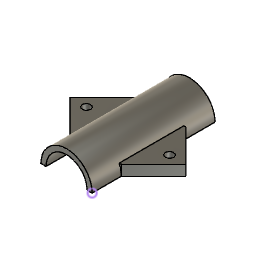
WhirlWax_Assem v1 (Autodesk Fusion 360 archive; units mm, degrees)
design "WeaponWireTunnel"
Autodesk Fusion 360 part; units mm, degrees
note: some values were not read from the file. Set by a fixed rule: which face or edge a step refers to.
sketch "Sketch1" plane through (0, 0, 0) normal (0, 1, 0) x (1, 0, 0)
  circle A0 centre (0, 0) radius 6.35
  circle A1 centre (0, 0) radius 7.9375
  line L0 (7.9375, 0.0011) -> (-7.9375, 0.0011)
  dimension "d1" = 12.7
  dimension "d2" = 15.875
  constraint coincident A0.centre A1.centre
  constraint concentric A0 A1
  constraint coincident A1 L0.start
  constraint coincident A1 L0.end
  constraint horizontal L0
  measures "d1" diameter of A0
  measures "d2" diameter of A1
extrude "Extrude1" add sketch "Sketch1" along normal blind 38.1 contours A0 A1 L0 picked at (7.3788, -0.3944) makes body 1
sketch "Sketch2" plane through (0, 0, 0) normal (0, 0, 1) x (1, 0, 0)
  line L0 (0, 1.0895) -> (-17.9605, 19.05)
  line L1 (-17.9605, 19.05) -> (0, 37.0105)
  line L2 (0, 37.0105) -> (17.9605, 19.05)
  line L3 (17.9605, 19.05) -> (0, 1.0895)
  line L4 (0, 1.0895) -> (0, 37.0105) construction
  line L5 (-17.9605, 19.05) -> (17.9605, 19.05) construction
  line L6 (7.9375, 0) -> (-7.9375, 0) construction
  line L7 (7.9375, 0) -> (7.9375, 38.1) construction
  line L8 (7.9375, 38.1) -> (-7.9375, 38.1) construction
  line L9 (-7.9375, 38.1) -> (-7.9375, 0) construction
  line L10 (0, 38.1) -> (0, 0) construction
  line L11 (-7.9375, 19.05) -> (7.9375, 19.05) construction
  circle A0 centre (-12.8805, 19.05) radius 1.27
  line L12 (-12.8805, 24.13) -> (-12.8805, 13.97) construction
  circle A1 centre (12.8805, 19.05) radius 1.27
  line L13 (7.9375, 9.027) -> (7.9375, 29.073)
  line L14 (-7.9375, 9.027) -> (-7.9375, 29.073)
  point P0 (0, 19.05)
  dimension "d5" = 25.4
  dimension "d6" = 25.4
  dimension "d7" = 2.54
  dimension "d9" = 5.08
  constraint perpendicular L0 L1
  constraint parallel L0 L2
  constraint parallel L1 L3
  constraint coincident L4 P0
  constraint coincident L5 P0
  constraint midpoint L8 L10.start
  constraint coincident L10.end origin
  constraint midpoint L9 L11.start
  constraint midpoint L7 L11.end
  constraint midpoint P0 L11
  constraint parallel L4 L10
  constraint coincident L5 A0.centre
  constraint coincident L1 L12.start
  constraint coincident L0 L12.end
  constraint perpendicular L5 L12
  constraint midpoint A0.centre L12
  constraint symmetric L10 A0 A1
  constraint coincident L7 L13.start
  constraint coincident L3 L13.start
  constraint coincident L2 L13.end
  constraint coincident L7 L13.end
  constraint coincident L9 L14.start
  constraint coincident L0 L14.start
  constraint coincident L9 L14.end
  constraint coincident L1 L14.end
  measures "d5" distance of L0.start L2.end
  measures "d6" distance of L1.end L2.end
  measures "d7" diameter of A0
  measures "d9" distance of L0.end L12
extrude "Extrude2" add sketch "Sketch2" along normal blind 3.175 separate body contours L0 L1 L14 | L2 L3 L13 makes body 2 at (9.1618, 19.05, 0) makes body 3 at (-9.1618, 19.05, 0)
extrude "Extrude3" add 1 faces at (-7.9375, 15.709, 1.0583) along direction (1, 0, 0) up to surface end surface at (7.9276, 25.4, 0.3957) on bodies 1 3 bodies 3 2 1
extrude "Extrude4" add 1 faces at (7.9375, 22.391, 2.1167) along direction (-1, 0, 0) up to surface end surface at (-6.8242, 15.709, 4.0539) on bodies 2 3 bodies 2 3
sketch "Sketch3" plane through (0, 0, 0) normal (0, 1, 0) x (1, 0, 0)
  point P0 (7.9375, 0.0011)

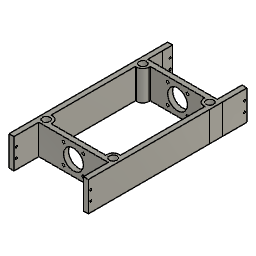
design "WhirlWax_Inside"
Autodesk Fusion 360 part; units mm, degrees
sketch "Sketch1" plane through (0, 0, 0) normal (0, 0, 1) x (1, 0, 0)
  line L0 (101.6, 0) -> (101.6, 203.2)
  line L1 (0, 203.2) -> (0, 0)
  line L2 (95.25, 27.3542) -> (95.25, 31.75)
  line L3 (95.25, 31.75) -> (6.35, 31.75)
  line L4 (6.35, 31.75) -> (6.35, 12.6739)
  line L5 (101.6, 31.75) -> (0, 31.75) construction
  line L6 (0, 31.75) -> (0, 47.625)
  line L7 (0, 47.625) -> (101.6, 47.625) construction
  line L8 (101.6, 47.625) -> (101.6, 31.75)
  circle A0 centre (7.9375, 39.6875) radius 7.9375 construction
  circle A1 centre (7.9375, 39.6875) radius 4.7625
  line L9 (50.8, 31.75) -> (50.8, 47.625)
  circle A2 centre (93.6625, 39.6875) radius 4.7625
  line L10 (0, 101.6) -> (101.6, 101.6)
  line L11 (101.6, 171.45) -> (0, 171.45) construction
  line L12 (95.25, 175.8458) -> (95.25, 171.45)
  line L13 (95.25, 171.45) -> (6.35, 171.45)
  line L14 (6.35, 171.45) -> (6.35, 190.5261)
  line L15 (101.6, 155.575) -> (101.6, 171.45)
  line L16 (0, 155.575) -> (101.6, 155.575) construction
  line L17 (0, 171.45) -> (0, 155.575)
  circle A3 centre (7.9375, 163.5125) radius 4.7625
  circle A4 centre (93.6625, 163.5125) radius 4.7625
  line L18 (95.25, 47.625) -> (6.35, 47.625)
  line L19 (6.35, 47.625) -> (6.35, 155.575)
  line L20 (6.35, 155.575) -> (95.25, 155.575)
  line L21 (95.25, 155.575) -> (95.25, 47.625)
  line L22 (6.35, 12.6739) -> (6.35, 0)
  line L23 (95.25, 27.3542) -> (95.25, 0)
  line L24 (0, 0) -> (6.35, 0)
  line L25 (95.25, 0) -> (101.6, 0)
  line L26 (6.35, 190.5261) -> (6.35, 203.2)
  line L27 (95.25, 175.8458) -> (95.25, 203.2)
  line L28 (101.6, 203.2) -> (95.25, 203.2)
  line L29 (6.35, 203.2) -> (0, 203.2)
  circle A5 centre (7.9375, 163.5125) radius 7.9375 construction
  circle A6 centre (93.6625, 163.5125) radius 7.9375 construction
  arc A7 (85.725, 163.5123) -> (93.6625, 155.575) centre (93.6625, 163.5125) ccw
  arc A8 (7.9421, 155.575) -> (15.875, 163.5125) centre (7.9375, 163.5125) ccw
  line L30 (85.8854, 165.1) -> (15.7146, 165.1) construction
  line L31 (15.875, 163.5125) -> (15.875, 165.1)
  line L32 (15.875, 165.1) -> (85.7183, 165.1)
  line L33 (85.7183, 165.1) -> (85.725, 163.5123)
  line L34 (15.875, 38.1) -> (85.7183, 38.1)
  line L35 (85.7183, 38.1) -> (85.725, 39.6877)
  line L36 (15.875, 39.6875) -> (15.875, 38.1)
  arc A9 (15.875, 39.6875) -> (7.9421, 47.625) centre (7.9375, 39.6875) ccw
  arc A10 (93.6625, 47.625) -> (85.725, 39.6877) centre (93.6625, 39.6875) ccw
  dimension "d1" = 101.6
  dimension "d2" = 203.2
  dimension "d4" = 6.35
  dimension "d5" = 6.35
  dimension "d7" = 15.875
  dimension "d8" = 9.525
  dimension "d10" = 6.35
  dimension "d11" = 6.35
  dimension "d23" = 31.75
  dimension "d24" = 6.35
  constraint horizontal L24
  constraint vertical L0
  constraint horizontal L28
  constraint vertical L1
  constraint coincident L1.end L24.start
  constraint vertical L2
  constraint horizontal L3
  constraint vertical L4
  constraint horizontal L5
  constraint vertical L6
  constraint horizontal L7
  constraint vertical L8
  constraint coincident L1 L6.end
  constraint coincident L0 L5.start
  constraint tangent L5 A0
  constraint tangent L7 A0
  constraint tangent L6 A0
  constraint concentric A0 A1
  constraint midpoint L5 L9.start
  constraint midpoint L7 L9.end
  constraint symmetric A1 L9 A2
  constraint midpoint L1 L10.start
  constraint midpoint L0 L10.end
  constraint symmetric L4.end L10 L14.end
  constraint symmetric L2.start L10 L12.start
  constraint symmetric L2.end L10 L12.end
  constraint symmetric L3.end L10 L13.end
  constraint symmetric L5.start L10 L11.start
  constraint symmetric L5.end L10 L11.end
  constraint symmetric L6.end L10 L16.start
  constraint symmetric L7.end L10 L15.start
  constraint symmetric A1 L10 A3
  constraint symmetric A2 L10 A4
  constraint horizontal L18
  constraint vertical L19
  constraint horizontal L20
  constraint vertical L21
  constraint coincident L16 L19.end
  constraint coincident L7 L18.start
  constraint coincident L2.end L5
  constraint perpendicular L22 L24
  constraint coincident L23.end L24
  constraint perpendicular L23 L24
  constraint collinear L24 L25
  constraint coincident L26.end L28
  constraint perpendicular L26 L28
  constraint perpendicular L27 L28
  constraint collinear L28 L29
  constraint tangent L13 A5
  constraint tangent L11 A6
  constraint coincident A6 A7.end
  constraint coincident L20 A7.end
  constraint coincident A4.centre A6.centre
  constraint coincident A5 A8.end
  constraint coincident A5 A8.start
  constraint coincident L20 A8.start
  constraint coincident A3.centre A5.centre
  constraint coincident A6 L30.start
  constraint coincident A5 L30.end
  constraint coincident L30 L31.end
  constraint perpendicular L30 L31
  constraint coincident L30 L32.end
  constraint symmetric L10 A7.start L35.end
  constraint symmetric L10 A7.end A10.start
  constraint symmetric L10 A7 A10
  constraint symmetric L10 A8.start A9.end
  constraint symmetric L10 A8.end L36.start
  constraint symmetric L10 A8 A9
  constraint symmetric L10 L31.end L34.start
  constraint symmetric L10 L32.end L34.end
  constraint coincident A2.centre A10.centre
  measures "d1" distance of L1.end L0.start
  measures "d2" distance of L1.end L1.start
  measures "d4" distance of L0 L2
  measures "d5" distance of L1 L4
  measures "d7" distance of L5 L7
  measures "d8" diameter of A1
  measures "d10" distance of L1 L19
  measures "d11" distance of L0 L21
  measures "d23" distance of L5 L22.end
  measures "d24" distance of L13 L30
extrude "Extrude1" add sketch "Sketch1" along normal blind 38.1 contours L0 L2 L3 L8 L9 L10 L18 L21 L23 L25 L34 L35 A10 | L0 L1 L10 L12 L13 L14 L15 L17 L19 L20 L21 L26 L27 L28 L29 A7 A8 L31 L32 L33 | L1 L3 L4 L6 L9 L10 L18 L19 L22 L24 L34 L36 A9
sketch "Sketch2" plane through (0, 155.575, 0) normal (0, -1, 0) x (1, 0, 0)
  line L0 (93.6625, 0) -> (95.25, 0)
  line L1 (95.25, 0) -> (95.25, 38.1)
  line L2 (95.25, 38.1) -> (93.6625, 38.1)
  line L3 (6.35, 38.1) -> (6.35, 0)
  circle A0 centre (63.4966, 31.75) radius 1.7272
  circle A1 centre (38.0966, 31.75) radius 1.7272
  circle A2 centre (38.0966, 6.35) radius 1.7272
  circle A3 centre (63.4966, 6.35) radius 1.7272
  circle A4 centre (50.7966, 19.05) radius 7.1 construction
  circle A5 centre (50.7966, 19.05) radius 12.7
  line L4 (93.6625, 38.1) -> (93.6625, 0)
  line L5 (6.35, 0) -> (7.9421, 0)
  line L6 (7.9421, 0) -> (7.9421, 38.1)
  line L7 (7.9421, 38.1) -> (6.35, 38.1)
  line L8 (15.875, 0) -> (85.7183, 0)
  line L9 (15.875, 38.1) -> (85.7183, 38.1)
  line L10 (63.4966, 31.75) -> (63.4966, 6.35) construction
  line L11 (63.4966, 6.35) -> (38.0966, 6.35) construction
  line L12 (38.0966, 6.35) -> (38.0966, 31.75) construction
  line L13 (38.0966, 31.75) -> (63.4966, 31.75) construction
  line L14 (50.7966, 38.1) -> (50.7966, 0)
  dimension "d18" = 25.4
  constraint concentric A4 A5
  constraint coincident A0.centre L10.start
  constraint coincident A3.centre L10.end
  constraint vertical L10
  constraint coincident A2.centre L11.end
  constraint perpendicular L10 L11
  constraint coincident A1.centre L12.end
  constraint perpendicular L11 L12
  constraint perpendicular L10 L13
  constraint tangent A5 L11
  constraint tangent A5 L10
  constraint tangent A5 L13
  constraint tangent A5 L12
  constraint midpoint L9 L14.start
  constraint midpoint L8 L14.end
  constraint coincident A4.centre L14
  measures "d18" diameter of A5
extrude "Extrude2" cut sketch "Sketch2" along normal up to surface (-15.875 mm away) and the other way up to surface (-123.825 mm away) contours A0 | A1 | A2 | A3 | A5 L14 | A5 L14
sketch "Sketch3" plane through (0, 0, 0) normal (-1, 0, 0) x (0, -1, 0)
  line L0 (-155.575, 0) -> (0, 0)
  line L1 (0, 0) -> (0, 38.1)
  line L2 (0, 38.1) -> (-155.575, 38.1)
  line L3 (-155.575, 38.1) -> (-155.575, 0)
  circle A0 centre (-3.175, 12.7) radius 1.27
  circle A1 centre (-3.175, 25.4) radius 1.27
  line L4 (-47.625, 38.1) -> (-155.575, 38.1)
  line L5 (-101.6, 38.1) -> (-101.6, 0)
  circle A2 centre (-200.025, 12.7) radius 1.27
  circle A3 centre (-200.025, 25.4) radius 1.27
  dimension "d25" = 2.54
  dimension "d26" = 2.54
  dimension "d27" = 12.7
  dimension "d28" = 12.7
  dimension "d29" = 3.175
  dimension "d30" = 3.175
  constraint midpoint L4 L5.start
  constraint coincident L0 L5.end
  constraint perpendicular L0 L5
  constraint symmetric A0 L5 A2
  constraint symmetric A1 L5 A3
  measures "d25" diameter of A0
  measures "d26" diameter of A1
  measures "d27" distance of L2 A1.centre
  measures "d28" distance of L0 A0.centre
  measures "d29" distance of L1 A0.centre
  measures "d30" distance of L1 A1.centre
extrude "Extrude3" cut sketch "Sketch3" along normal through all and the other way through all contours A0 | A1 | A2 | A3
sketch "Sketch4" plane through (0, 38.1, 0) normal (0, 1, 0) x (-1, 0, 0)
  circle A0 centre (-50.7966, 19.05) radius 12.7
  circle A1 centre (-38.0966, 6.35) radius 1.7272
  circle A2 centre (-63.4966, 31.75) radius 1.7272
  circle A3 centre (-38.0966, 31.75) radius 1.7272
  circle A4 centre (-63.4966, 6.35) radius 1.7272
  line L0 (-85.7183, 0) -> (-15.875, 0)
  line L1 (-15.875, 0) -> (-15.875, 38.1)
  line L2 (-15.875, 38.1) -> (-85.7183, 38.1)
  line L3 (-85.7183, 38.1) -> (-85.7183, 0)
  line L4 (-95.25, 0) -> (-95.25, 38.1)
  circle A5 centre (-86.36, 0) radius 5.715
  circle A6 centre (-86.36, 0) radius 8.89
  circle A7 centre (-50.7966, 19.05) radius 30.1625 construction
  dimension "d33" = 17.78
  dimension "d34" = 60.325
  dimension "d35" = 11.43
  constraint coincident L0 A5.centre
  constraint concentric A5 A6
  constraint concentric A0 A7
  constraint tangent L4 A6
  measures "d33" diameter of A6
  measures "d34" diameter of A7
  measures "d35" diameter of A5
extrude "Extrude4" cut sketch "Sketch4" against normal blind 6.35 contours L0 L3 A5 picked at (-85.4455, 3.7347)
equation "d34 = 2 in + ( 3 / 8 ) * 1 in"

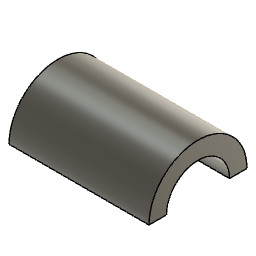
design "lilTunnel"
Autodesk Fusion 360 part; units mm, degrees
sketch "Sketch1" plane through (0, 0, 0) normal (1, 0, 0) x (0, 1, 0)
  line L0 (0, 0) -> (101.6, 0) construction
  line L1 (101.6, 0) -> (101.6, 38.1) construction
  line L2 (101.6, 38.1) -> (0, 38.1) construction
  line L3 (0, 38.1) -> (0, 0) construction
  circle A0 centre (50.8, 19.05) radius 30.1625 construction
  line L4 (101.6, 0) -> (85.725, 0) construction
  line L5 (85.725, 15.875) -> (101.6, 15.875) construction
  line L6 (101.6, 15.875) -> (101.6, 0) construction
  arc A1 (86.36, 5.715) -> (80.645, 0) centre (86.36, 0) ccw
  arc A2 (86.36, 8.89) -> (77.47, 0) centre (86.36, 0) ccw
  line L7 (86.36, 8.89) -> (86.36, 5.715)
  line L8 (77.47, 0) -> (80.645, 0)
  line L9 (101.6, 38.1) -> (95.25, 38.1) construction
  line L10 (95.25, 38.1) -> (95.25, -0.2036) construction
  line L11 (95.25, -0.2036) -> (101.6, -0.2036) construction
  line L12 (101.6, -0.2036) -> (101.6, 38.1) construction
  arc A3 (92.075, 0) -> (86.36, 5.715) centre (86.36, 0) ccw
  arc A4 (95.25, 0) -> (86.36, 8.89) centre (86.36, 0) ccw
  line L13 (92.075, 0) -> (95.25, 0)
  dimension "d1" = 101.6
  dimension "d2" = 38.1
  dimension "d3" = 60.325
  dimension "d4" = 15.875
  dimension "d5" = 15.875
  dimension "d8" = 6.35
  dimension "d12" = 50.8
  dimension "d13" = 5.715
  dimension "d14" = 8.89
  constraint horizontal L0
  constraint vertical L1
  constraint horizontal L2
  constraint vertical L3
  constraint coincident L0.start L3.end
  constraint horizontal L4
  constraint horizontal L5
  constraint vertical L6
  constraint coincident L0 A1.end
  constraint coincident L0 A2.end
  constraint horizontal L9
  constraint vertical L10
  constraint horizontal L11
  constraint vertical L12
  constraint coincident L10 A4.start
  measures "d1" distance of L0.start L0.end
  measures "d2" distance of L0.start L2.end
  measures "d3" diameter of A0
  measures "d4" distance of L0.end L4.end
  measures "d5" distance of L0.end L5.end
  measures "d8" distance of L1.end L9.end
  measures "d12" distance of L3 A0.centre
  measures "d13" radius of A3
  measures "d14" radius of A4
extrude "Extrude1" add sketch "Sketch1" along normal blind 25.4
equation "d3 = 2 3/8\""

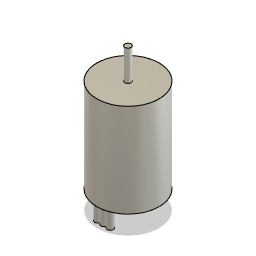
design "2030 motor"
Autodesk Fusion 360 part; units mm, degrees
sketch "Sketch1" plane through (0, 0, 0) normal (0, 1, 0) x (1, 0, 0)
  circle A0 centre (0, -2.6241) radius 10
  dimension "d1" = 20
  measures "d1" diameter of A0
extrude "Extrude1" add sketch "Sketch1" along normal blind 30 makes body 1
sketch "Sketch2" plane through (0, 30, 0) normal (0, 1, 0) x (-1, 0, 0)
  circle A0 centre (0, 2.6241) radius 10
  circle A1 centre (0, 2.6241) radius 1
  dimension "d4" = 2
  constraint concentric A0 A1
  measures "d4" diameter of A1
extrude "Extrude2" add sketch "Sketch2" along normal blind 9.8 contours A1 bodies 1
sketch "Sketch3" plane through (0, 0, 0) normal (0, -1, 0) x (1, 0, 0)
  circle A0 centre (0, 2.6241) radius 10
  circle A1 centre (-2, 10.3376) radius 1
  circle A2 centre (0, 10.3376) radius 1
  circle A3 centre (2, 10.3376) radius 1
  dimension "d7" = 2
  dimension "d8" = 2
  dimension "d9" = 2
  dimension "d10" = 2
  dimension "d11" = 2
  constraint horizontal A2.centre A3.centre
  constraint horizontal A1.centre A2.centre
  measures "d7" diameter of A1
  measures "d8" diameter of A2
  measures "d9" diameter of A3
  measures "d10" distance of A1.centre A2.centre
  measures "d11" distance of A2.centre A3.centre
extrude "Extrude3" add sketch "Sketch3" along normal blind 6 separate body contours A1 | A3 | A2 makes body 2
combine "Combine1" operation add target body 2 tool bodies 1

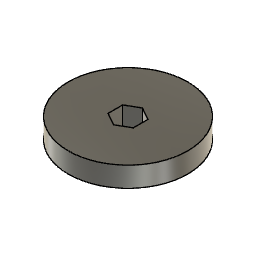
design "Basic_Wheel"
Autodesk Fusion 360 part; units mm, degrees
sketch "Sketch1" plane through (0, 0, 0) normal (0, 0, 1) x (1, 0, 0)
  circle A0 centre (0, 0) radius 30.1625
  line L0 (6.35, 3.6662) -> (0, 7.3323)
  line L1 (0, 7.3323) -> (-6.35, 3.6662)
  line L2 (-6.35, 3.6662) -> (-6.35, -3.6662)
  line L3 (-6.35, -3.6662) -> (0, -7.3323)
  line L4 (0, -7.3323) -> (6.35, -3.6662)
  line L5 (6.35, -3.6662) -> (6.35, 3.6662)
  dimension "d1" = 60.325
  dimension "d5" = 6.35
  constraint coincident A0.centre origin
  measures "d1" diameter of A0
  measures "d5" distance of A0.centre L5
extrude "Extrude1" add sketch "Sketch1" along normal blind 10.16
equation "d1 = 2 in + ( 3 / 8 ) * 1 in"

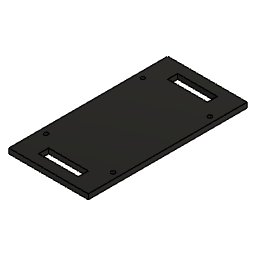
design "WhirlWax_TopPlate"
Autodesk Fusion 360 part; units mm, degrees
sketch "Sketch1" plane through (0, 0, 0) normal (0, 0, 1) x (1, 0, 0)
  line L0 (101.6, 203.2) -> (0, 203.2)
  line L1 (101.6, 203.2) -> (101.6, 0)
  line L2 (0, 0) -> (0, 203.2)
  line L3 (0, 0) -> (101.6, 0)
  dimension "d37" = 203.2
  dimension "d38" = 101.6
  constraint horizontal L0
  constraint perpendicular L0 L2
  constraint coincident L2.start L3.start
  constraint perpendicular L1 L3
  constraint parallel L0 L3
  measures "d37" distance of L0.end L2.start
  measures "d38" distance of L2.start L1.end
extrude "Extrude1" add sketch "Sketch1" along normal blind 6.35
sketch "Sketch2" plane through (0, 0, 0) normal (0, 1, 0) x (1, 0, 0)
  line L0 (0, -3.175) -> (76.2, -3.175) construction
  line L1 (76.2, -3.175) -> (76.2, -41.275) construction
  line L2 (76.2, -41.275) -> (0, -41.275) construction
  line L3 (0, -41.275) -> (0, -3.175) construction
  line L4 (38.1, -41.275) -> (38.1, -3.175) construction
  line L5 (76.2, -22.225) -> (0, -22.225) construction
  circle A0 centre (38.1, -22.225) radius 23.8125
  point P0 (101.6, -6.35)
  dimension "d6" = 47.625
  dimension "d32" = 38.1
  constraint horizontal L0
  constraint vertical L1
  constraint horizontal L2
  constraint vertical L3
  constraint midpoint L2 L4.start
  constraint midpoint L0 L4.end
  constraint midpoint L1 L5.start
  constraint midpoint L3 L5.end
  constraint midpoint L4 A0.centre
  measures "d6" diameter of A0
  measures "d32" distance of L0.end L1.end
sketch "Sketch3" plane through (0, 0, 6.35) normal (0, 0, 1) x (-1, 0, 0)
  line L0 (-101.6, 0) -> (-101.6, -203.2)
  line L1 (0, -203.2) -> (0, 0)
  line L2 (0, 0) -> (-101.6, 0) construction
  line L3 (-61.9125, 0) -> (-14.2875, 0) construction
  line L4 (0, -31.75) -> (-101.6, -31.75)
  line L5 (-101.6, -31.75) -> (-101.6, -47.625)
  line L6 (-101.6, -47.625) -> (0, -47.625)
  line L7 (0, -47.625) -> (0, -31.75)
  circle A0 centre (-93.6625, -39.6875) radius 7.9375 construction
  circle A1 centre (-93.6625, -39.6875) radius 4.7625
  circle A2 centre (-93.6625, -39.6875) radius 2.54
  line L8 (-50.8, -203.2) -> (-50.8, 0) construction
  line L9 (-50.8, -101.6) -> (-8.4033, -101.6)
  line L10 (-101.6, -155.575) -> (0, -155.575)
  line L11 (0, -171.45) -> (-101.6, -171.45)
  circle A3 centre (-93.6625, -163.5125) radius 4.7625
  line L12 (-101.6, -171.45) -> (-101.6, -155.575)
  line L13 (0, -155.575) -> (0, -171.45)
  circle A4 centre (-93.6625, -163.5125) radius 2.54
  line L14 (-25.4, -190.5) -> (-76.2, -190.5)
  line L15 (-76.2, -190.5) -> (-76.2, -177.8)
  line L16 (-76.2, -177.8) -> (-25.4, -177.8)
  line L17 (-25.4, -177.8) -> (-25.4, -190.5)
  line L18 (0, 0) -> (-101.6, 0)
  circle A5 centre (-7.9375, -163.5125) radius 4.7625
  circle A6 centre (-7.9375, -163.5125) radius 2.54
  circle A7 centre (-7.9375, -39.6875) radius 4.7625
  circle A8 centre (-7.9375, -39.6875) radius 2.54
  line L19 (-76.2, -12.7) -> (-76.2, -25.4)
  line L20 (-76.2, -25.4) -> (-25.4, -25.4)
  line L21 (-25.4, -12.7) -> (-76.2, -12.7)
  line L22 (-25.4, -25.4) -> (-25.4, -12.7)
  line L23 (-101.6, -203.2) -> (0, -203.2)
  point P0 (-93.6625, -163.5125)
  dimension "d25" = 15.875
  dimension "d26" = 9.525
  dimension "d27" = 5.08
  dimension "d29" = 12.7
  dimension "d30" = 25.4
  dimension "d31" = 25.4
  dimension "d36" = 6.35
  dimension "d39" = 12.7
  constraint coincident L1.end L2.start
  constraint coincident L0.start L2.end
  constraint horizontal L4
  constraint vertical L5
  constraint horizontal L6
  constraint vertical L7
  constraint coincident L1 L4.start
  constraint tangent L4 A0
  constraint tangent L5 A0
  constraint tangent L6 A0
  constraint concentric A0 A1
  constraint concentric A1 A2
  constraint midpoint L8 L9.start
  constraint symmetric L4.start L9 L11.start
  constraint symmetric L4.end L9 L11.end
  constraint symmetric L5.end L9 L10.start
  constraint symmetric L6.end L9 L10.end
  constraint symmetric A1 L9 A3
  constraint symmetric A0.centre L9 P0
  constraint symmetric A2 L9 A4
  constraint horizontal L14
  constraint vertical L15
  constraint horizontal L16
  constraint vertical L17
  constraint coincident L0 L5.end
  constraint horizontal L9
  constraint symmetric A1 L8 A7
  constraint symmetric A2 L8 A8
  constraint symmetric L8 A3 A5
  constraint symmetric L8 A4 A6
  constraint symmetric L9 L14.start L21.start
  constraint symmetric L9 L14.end L19.start
  constraint symmetric L9 L15.end L19.end
  constraint symmetric L9 L16.end L20.end
  constraint midpoint L18 L8.end
  constraint midpoint L8.start L23
  measures "d25" distance of L4.start L6.end
  measures "d26" diameter of A1
  measures "d27" diameter of A2
  measures "d29" distance of L14.start L16.end
  measures "d30" distance of L1 L17
  measures "d31" distance of L0 L15
  measures "d36" distance of L11 L16
  measures "d39" distance of L14 L23
extrude "Extrude6" cut sketch "Sketch3" along normal through all and the other way through all contours A2 | A4 | L14 L15 L16 L17 | A6 | A8 | L19 L20 L21 L22
equation "d6 = 1 in + ( 7 / 8 ) * 1 in"

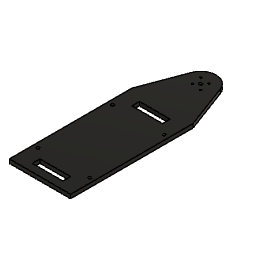
design "WhirlWax_Plate_D3536"
Autodesk Fusion 360 part; units mm, degrees
sketch "Sketch1" plane through (0, 0, 0) normal (0, 0, 1) x (1, 0, 0)
  line L0 (101.6, 203.2) -> (0, 203.2)
  line L1 (101.6, 203.2) -> (101.6, 0)
  line L2 (0, 0) -> (0, 203.2)
  line L3 (0, 0) -> (101.6, 0)
  dimension "d37" = 203.2
  dimension "d38" = 101.6
  constraint horizontal L0
  constraint perpendicular L0 L2
  constraint coincident L2.start L3.start
  constraint perpendicular L1 L3
  constraint parallel L0 L3
  measures "d37" distance of L0.end L2.start
  measures "d38" distance of L2.start L1.end
extrude "Extrude1" add sketch "Sketch1" along normal blind 6.35
sketch "Sketch2" plane through (0, 0, 0) normal (0, 1, 0) x (1, 0, 0)
  line L0 (0, -3.175) -> (76.2, -3.175) construction
  line L1 (76.2, -3.175) -> (76.2, -41.275) construction
  line L2 (76.2, -41.275) -> (0, -41.275) construction
  line L3 (0, -41.275) -> (0, -3.175) construction
  line L4 (38.1, -41.275) -> (38.1, -3.175) construction
  line L5 (76.2, -22.225) -> (0, -22.225) construction
  circle A0 centre (38.1, -22.225) radius 23.8125
  point P0 (101.6, -6.35)
  dimension "d6" = 47.625
  dimension "d32" = 38.1
  constraint horizontal L0
  constraint vertical L1
  constraint horizontal L2
  constraint vertical L3
  constraint midpoint L2 L4.start
  constraint midpoint L0 L4.end
  constraint midpoint L1 L5.start
  constraint midpoint L3 L5.end
  constraint midpoint L4 A0.centre
  measures "d6" diameter of A0
  measures "d32" distance of L0.end L1.end
sketch "Sketch3" plane through (0, 0, 6.35) normal (0, 0, 1) x (-1, 0, 0)
  line L0 (-101.6, 0) -> (-101.6, -203.2)
  line L1 (0, -203.2) -> (0, 0)
  line L2 (0, 0) -> (-101.6, 0) construction
  line L3 (-61.9125, 0) -> (-14.2875, 0) construction
  line L4 (0, -31.75) -> (-101.6, -31.75)
  line L5 (-101.6, -31.75) -> (-101.6, -47.625)
  line L6 (-101.6, -47.625) -> (0, -47.625)
  line L7 (0, -47.625) -> (0, -31.75)
  circle A0 centre (-93.6625, -39.6875) radius 7.9375 construction
  circle A1 centre (-93.6625, -39.6875) radius 4.7625
  circle A2 centre (-93.6625, -39.6875) radius 2.54
  line L8 (-50.8, -203.2) -> (-50.8, 0) construction
  line L9 (-50.8, -101.6) -> (-8.4033, -101.6)
  line L10 (-101.6, -155.575) -> (0, -155.575)
  line L11 (0, -171.45) -> (-101.6, -171.45)
  circle A3 centre (-93.6625, -163.5125) radius 4.7625
  line L12 (-101.6, -171.45) -> (-101.6, -155.575)
  line L13 (0, -155.575) -> (0, -171.45)
  circle A4 centre (-93.6625, -163.5125) radius 2.54
  line L14 (-25.4, -190.5) -> (-76.2, -190.5)
  line L15 (-76.2, -190.5) -> (-76.2, -177.8)
  line L16 (-76.2, -177.8) -> (-25.4, -177.8)
  line L17 (-25.4, -177.8) -> (-25.4, -190.5)
  line L18 (0, 0) -> (-101.6, 0)
  circle A5 centre (-7.9375, -163.5125) radius 4.7625
  circle A6 centre (-7.9375, -163.5125) radius 2.54
  circle A7 centre (-7.9375, -39.6875) radius 4.7625
  circle A8 centre (-7.9375, -39.6875) radius 2.54
  line L19 (-76.2, -12.7) -> (-76.2, -25.4)
  line L20 (-76.2, -25.4) -> (-25.4, -25.4)
  line L21 (-25.4, -12.7) -> (-76.2, -12.7)
  line L22 (-25.4, -25.4) -> (-25.4, -12.7)
  line L23 (-101.6, -203.2) -> (0, -203.2)
  point P0 (-93.6625, -163.5125)
  dimension "d25" = 15.875
  dimension "d26" = 9.525
  dimension "d27" = 5.08
  dimension "d29" = 12.7
  dimension "d30" = 25.4
  dimension "d31" = 25.4
  dimension "d36" = 6.35
  dimension "d39" = 12.7
  constraint coincident L1.end L2.start
  constraint coincident L0.start L2.end
  constraint horizontal L4
  constraint vertical L5
  constraint horizontal L6
  constraint vertical L7
  constraint coincident L1 L4.start
  constraint tangent L4 A0
  constraint tangent L5 A0
  constraint tangent L6 A0
  constraint concentric A0 A1
  constraint concentric A1 A2
  constraint midpoint L8 L9.start
  constraint symmetric L4.start L9 L11.start
  constraint symmetric L4.end L9 L11.end
  constraint symmetric L5.end L9 L10.start
  constraint symmetric L6.end L9 L10.end
  constraint symmetric A1 L9 A3
  constraint symmetric A0.centre L9 P0
  constraint symmetric A2 L9 A4
  constraint horizontal L14
  constraint vertical L15
  constraint horizontal L16
  constraint vertical L17
  constraint coincident L0 L5.end
  constraint horizontal L9
  constraint symmetric A1 L8 A7
  constraint symmetric A2 L8 A8
  constraint symmetric L8 A3 A5
  constraint symmetric L8 A4 A6
  constraint symmetric L9 L14.start L21.start
  constraint symmetric L9 L14.end L19.start
  constraint symmetric L9 L15.end L19.end
  constraint symmetric L9 L16.end L20.end
  constraint midpoint L18 L8.end
  constraint midpoint L8.start L23
  measures "d25" distance of L4.start L6.end
  measures "d26" diameter of A1
  measures "d27" diameter of A2
  measures "d29" distance of L14.start L16.end
  measures "d30" distance of L1 L17
  measures "d31" distance of L0 L15
  measures "d36" distance of L11 L16
  measures "d39" distance of L14 L23
extrude "Extrude6" cut sketch "Sketch3" along normal through all and the other way through all contours A2 | A4 | L14 L15 L16 L17 | A6 | A8 | L19 L20 L21 L22
sketch "Sketch5" plane through (0, 0, 6.35) normal (0, 0, 1) x (-1, 0, 0)
  circle A0 centre (-93.6625, -39.6875) radius 2.54
  circle A1 centre (-93.6625, -163.5125) radius 2.54
  circle A2 centre (-7.9375, -39.6875) radius 2.54
  circle A3 centre (-7.9375, -163.5125) radius 2.54
  line L0 (-25.4, -177.8) -> (-25.4, -190.5)
  line L1 (-25.4, -190.5) -> (-76.2, -190.5)
  line L2 (-76.2, -190.5) -> (-76.2, -177.8)
  line L3 (-76.2, -177.8) -> (-25.4, -177.8)
  line L4 (-25.4, -25.4) -> (-76.2, -25.4)
  line L5 (-76.2, -25.4) -> (-76.2, -12.7)
  line L6 (-76.2, -12.7) -> (-25.4, -12.7)
  line L7 (-25.4, -12.7) -> (-25.4, -25.4)
  line L8 (-101.6, -203.2) -> (0, -203.2)
  line L9 (0, -203.2) -> (0, 0)
  line L10 (0, 0) -> (-101.6, 0)
  line L11 (-101.6, 0) -> (-101.6, -203.2)
  line L12 (-50.8, -203.2) -> (-50.8, -292.1) construction
  circle A4 centre (-50.8, -266.7) radius 25.4
  line L13 (-101.6, -203.2) -> (-74.5978, -275.5783)
  line L14 (0, -203.2) -> (-27.0022, -275.5783)
  circle A5 centre (-44.0825, -259.9825) radius 1.5
  circle A6 centre (-57.5175, -273.4175) radius 1.5
  line L15 (-57.5175, -273.4175) -> (-44.0825, -259.9825) construction
  circle A7 centre (-41.9612, -275.5388) radius 1.5
  circle A8 centre (-59.6388, -257.8612) radius 1.5
  line L16 (-41.9612, -275.5388) -> (-59.6388, -257.8612) construction
  circle A9 centre (-50.8, -266.7) radius 2.54
  point P0 (-50.8, -266.7)
  dimension "d40" = 25.4
  dimension "d43" = 3
  dimension "d44" = 3
  dimension "d45" = 19
  dimension "d46" = 3
  dimension "d47" = 3
  dimension "d48" = 25
  dimension "d49" = 135
  dimension "d52" = 63.5
  constraint midpoint L8 L12.start
  constraint perpendicular L8 L12
  constraint coincident L12 P0
  constraint coincident L12.end A4
  constraint coincident L8.start L11.end
  constraint coincident A4 L13.end
  constraint tangent A4 L13
  constraint coincident L8.end L9.start
  constraint coincident A4 L14.end
  constraint tangent A4 L14
  constraint coincident A6.centre L15.start
  constraint coincident A5.centre L15.end
  constraint coincident A7.centre L16.start
  constraint coincident A8.centre L16.end
  constraint perpendicular L15 L16
  constraint midpoint L15 L16
  constraint midpoint L16 P0
  constraint coincident P0 A4.centre
  measures "d40" distance of L12.end P0
  measures "d43" diameter of A5
  measures "d44" diameter of A6
  measures "d45" distance of A6.centre A5.centre
  measures "d46" diameter of A7
  measures "d47" diameter of A8
  measures "d48" distance of A7.centre A8.centre
  measures "d49" angle of L12 L16
  measures "d52" distance of L12.start P0
extrude "Extrude7" add sketch "Sketch5" against normal blind 6.35 contours L8 A4 L13 L14 | A4
equation "d6 = 1 in + ( 7 / 8 ) * 1 in"

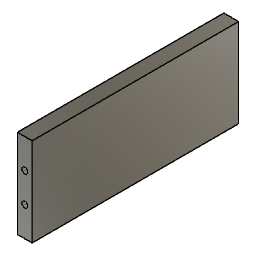
design "WhirlWax_WheelGuardNoTunnel"
Autodesk Fusion 360 part; units mm, degrees
sketch "Sketch1" plane through (0, 0, 0) normal (1, 0, 0) x (0, 1, 0)
  line L0 (0, 0) -> (88.9, 0)
  line L1 (88.9, 0) -> (88.9, 38.1)
  line L2 (88.9, 38.1) -> (0, 38.1)
  line L3 (0, 38.1) -> (0, 0)
  dimension "d1" = 88.9
  dimension "d2" = 38.1
  constraint horizontal L0
  constraint vertical L1
  constraint horizontal L2
  constraint vertical L3
  constraint coincident L0.start L3.end
  measures "d1" distance of L0.start L0.end
  measures "d2" distance of L0.start L2.end
extrude "Extrude1" add sketch "Sketch1" along normal blind 6.35
sketch "Sketch2" plane through (0, 0, 0) normal (0, -1, 0) x (1, 0, 0)
  line L0 (0, 38.1) -> (0, 0)
  line L1 (0, 0) -> (6.35, 0)
  line L2 (6.35, 0) -> (6.35, 38.1)
  line L3 (6.35, 38.1) -> (0, 38.1)
  line L4 (3.175, 38.1) -> (3.175, 0) construction
  circle A0 centre (3.175, 25.4) radius 1.27
  circle A1 centre (3.175, 12.7) radius 1.27
  dimension "d5" = 2.54
  dimension "d6" = 2.54
  dimension "d7" = 12.7
  dimension "d8" = 12.7
  constraint midpoint L3 L4.start
  constraint midpoint L1 L4.end
  constraint coincident L4 A0.centre
  constraint coincident L4 A1.centre
  measures "d5" diameter of A0
  measures "d6" diameter of A1
  measures "d7" distance of L1 A1.centre
  measures "d8" distance of L3 A0.centre
extrude "Extrude2" cut sketch "Sketch2" along normal through all and the other way through all contours A0 | A1

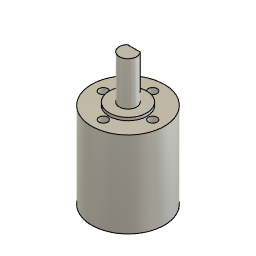
design "25mm gearbox"
Autodesk Fusion 360 part; units mm, degrees
sketch "Sketch1" plane through (0, 0, 0) normal (0, 1, 0) x (1, 0, 0)
  circle A0 centre (0, 0) radius 12.5
  circle A1 centre (0, 0) radius 3
  circle A2 centre (0, 0) radius 6.5
  circle A3 centre (0, 0) radius 8.5 construction
  circle A4 centre (0, -8.5) radius 1.5
  circle A5 centre (8.5, 0) radius 1.5
  circle A6 centre (0, 8.5) radius 1.5
  circle A7 centre (-8.5, 0) radius 1.5
  dimension "d1" = 25
  dimension "d2" = 6
  dimension "d3" = 13
  dimension "d10" = 17
  dimension "d11" = 3
  dimension "d13" = 360
  constraint coincident A0.centre A1.centre
  constraint concentric A0 A1
  constraint concentric A1 A2
  constraint coincident A3 A4.centre
  constraint vertical A0.centre A4.centre
  measures "d1" diameter of A0
  measures "d2" diameter of A1
  measures "d3" diameter of A2
  measures "d10" diameter of A3
  measures "d11" diameter of A4
extrude "Extrude1" add sketch "Sketch1" along normal blind 29.5 contours A0 | A1 | A2 | A4 | A5 | A6 | A7
extrude "Extrude2" add sketch "Sketch1" along normal blind 30.5 contours A2
extrude "Extrude3" add sketch "Sketch1" along normal blind 45.5 contours A1
extrude "Extrude4" cut sketch "Sketch1" along normal blind 9.5001 from surface at 20 contours A4 | A5 | A6 | A7
sketch "Sketch2" plane through (0, 45.5, 0) normal (0, 1, 0) x (-1, 0, 0)
  circle A0 centre (0, 0) radius 3
  line L0 (2.1979, 3) -> (-2.9389, 3)
  line L1 (2.2361, -2) -> (-2.2361, -2)
  dimension "d17" = 5
  constraint tangent A0 L0
  constraint horizontal L0
  constraint coincident A0 L1.start
  constraint coincident A0 L1.end
  constraint horizontal L1
  measures "d17" distance of L0 L1
extrude "Extrude5" cut sketch "Sketch2" against normal blind 12 contours A0 L1 picked at (-0.6449, -2.0976)
